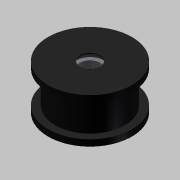
# Autodesk Inventor part: MSK01-06A
Saved by Autodesk Inventor 2012 SP1 (Build 160190100, 190)
## iProperties
Created: 2012-01-26
Part Number: MSK01-06A
Document SubType Name: Modeling
Designer: ERF
Density: 1 g/cm^3
Mass: 2.33537 g
Surface Area: 50.9321 cm^2
Volume: 1.82508 cm^3
Description: smooth idler assembly
Material: Default
Stock Number: B30041
Vendor: buildlog.net
Project: Shapeoko
Author: ERF
Title: Smooth Idler Assembly
Autodesk Inventor part; units mm, degrees
ref_plane "YZ Plane" through (0, 0, 0) normal (1, 0, 0) x (0, 1, 0)
ref_plane "XZ Plane" through (0, 0, 0) normal (0, 1, 0) x (-1, 0, 0)
ref_plane "XY Plane" through (0, 0, 0) normal (0, 0, 1) x (1, 0, 0)
sketch "Sketch1" plane through (0, 10.1, 0) normal (0, 1, 0) x (1, 0, 0)
  circle A0 centre (0, 0) radius 2.5 projected
  circle A1 centre (0, 0) radius 10.5 projected
  circle A2 centre (0, 0) radius 3.175
  dimension "d1" = 6.35
  constraints: 1 centre point, 1 coincident
  measures "d1" diameter of A2
extrude "Extrusion1" add sketch "Sketch1" against normal blind 0.00254 contours A2
sketch "Sketch2" plane through (0, 10.1, 0) normal (0, 1, 0) x (1, 0, 0)
  circle A0 centre (0, 0) radius 2.5 projected
  circle A1 centre (0, 0) radius 10.5 projected
extrude "Extrusion2" add sketch "Sketch2" along normal blind 0.00254
body "Solid1"
body "Srf1"
